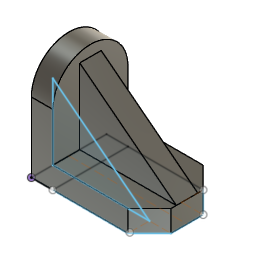
A1 (Autodesk Fusion 360 design; units mm, degrees)
Autodesk Fusion 360 part; units mm, degrees
sketch "Base" plane through (0, 0, 0) normal (0, 0, 1) x (1, 0, 0)
  line L0 (0, 0) -> (12, 0)
  line L1 (12, 0) -> (12, 42)
  line L2 (12, 42) -> (0, 42)
  line L3 (0, 42) -> (0, 0)
  line L4 (12, 42) -> (54, 42)
  line L5 (54, 0) -> (12, 0)
  line L6 (54, 0) -> (54, 1) construction
  line L7 (54, 0) -> (54, 12) construction
  line L8 (54, 12) -> (66, 12) construction
  line L9 (66, 12) -> (54, 0)
  line L10 (66, 12) -> (66, 30)
  line L11 (0, 21) -> (66, 21) construction
  line L12 (54, 30) -> (66, 30) construction
  line L13 (54, 42) -> (54, 30) construction
  line L14 (66, 30) -> (54, 42)
  dimension "d1" = 12
  dimension "d2" = 42
  dimension "d4" = 18
  constraint horizontal L0
  constraint vertical L1
  constraint horizontal L2
  constraint vertical L3
  constraint coincident L0.start L3.end
  constraint horizontal L4
  constraint horizontal L5
  constraint perpendicular L5 L7
  constraint perpendicular L8 L10
  constraint midpoint L3 L11.start
  constraint midpoint L10 L11.end
  constraint symmetric L5.start L11 L4.end
  constraint symmetric L7.end L11 L12.start
  constraint symmetric L8.end L11 L10.end
  measures "d1" distance of L0.start L0.end
  measures "d2" distance of L0.start L2.end
  measures "d4" distance of L8.end L10.end
extrude "Extrude1" add sketch "Base" along normal blind 12 contours L1 L4 L5 L9 L10 L14
extrude "Extrude2" add sketch "Base" along normal blind 60 contours L0 L1 L2 L3
fillet "Fillet1" radius 21 2 edges at (6, 0, 60) (6, 42, 60)
sketch "Triangle" plane through (0, 0, 0) normal (0, 1, 0) x (1, 0, 0)
  line L0 (12, -12) -> (12, -54)
  line L1 (12, -12) -> (66, -12)
  line L2 (66, -12) -> (12, -54)
  constraint vertical L0
  constraint perpendicular L0 L1
extrude "Extrude3" add sketch "Triangle" along normal blind 12 from surface at 15
named bodies: "MainBodyA1"
